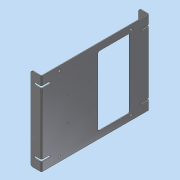
# Autodesk Inventor part: Innengehäuse gebogen
Saved by Autodesk Inventor 2015 SP1 (Build 190203100, 203)
## iProperties
Created: 2015-04-14
Part Number: Innengehäuse gebogen
Material: Stahl AISI 1015
Document SubType Name: Modeling
Designer: ElMatinho
Density: 7.87 g/cm^3
Appearance: Stahl
Author: ElMatinho
Autodesk Inventor part; units mm, degrees
ref_plane "YZ Plane" through (0, 0, 0) normal (1, 0, 0) x (0, 1, 0)
ref_plane "XZ Plane" through (0, 0, 0) normal (0, 1, 0) x (-1, 0, 0)
ref_plane "XY Plane" through (0, 0, 0) normal (0, 0, 1) x (1, 0, 0)
sketch "Skizze1" plane through (0, 0, 0) normal (0, 0, 1) x (1, 0, 0)
  line L0 (-65.8319, 0) -> (313.5681, 0) projected
  line L1 (0, -176.4249) -> (0, 176.4249) projected
  line L2 (13.3681, -123) -> (13.3681, 123)
  line L3 (13.3681, -125.5) -> (259.3681, -125.5) construction
  line L4 (10.8681, 125.5) -> (-11.6319, 125.5)
  line L5 (-11.6319, 125.5) -> (-11.6319, 104.5)
  line L6 (10.8681, -125.5) -> (-11.6319, -125.5)
  line L7 (13.3681, -125.5) -> (35.8681, -125.5) construction
  line L8 (-11.6319, -125.5) -> (-11.6319, -124)
  line L9 (-11.6319, -124) -> (10.8681, -124)
  line L10 (11.8681, -123) -> (11.8681, 123)
  line L11 (10.8681, 124) -> (-10.1319, 124)
  line L12 (-10.1319, 124) -> (-10.1319, 104.5)
  line L13 (-10.1319, 104.5) -> (-11.6319, 104.5)
  arc A0 (13.3681, 123) -> (10.8681, 125.5) centre (10.8681, 123) ccw
  arc A1 (10.8681, -125.5) -> (13.3681, -123) centre (10.8681, -123) ccw
  arc A2 (10.8681, -124) -> (11.8681, -123) centre (10.8681, -123) ccw
  arc A3 (11.8681, 123) -> (10.8681, 124) centre (10.8681, 123) ccw
  point P0 (0, 0)
  point P1 (13.3681, 125.5)
  point P2 (11.8681, -124)
  point P3 (11.8681, 124)
  dimension "d0" = 251
  dimension "d1" = 90
  dimension "d2" = 25
  dimension "d3" = 90
  dimension "d4" = 21
  dimension "d5" = 90
  dimension "d6" = 25
  dimension "d7" = 180
  dimension "d8" = 1.5
  dimension "d9" = 90
  dimension "d10" = 23.5
  dimension "d11" = 90
  dimension "d12" = 248
  dimension "d13" = 90
  dimension "d14" = 22
  dimension "d15" = 90
  dimension "d17" = 1
  constraints: 24 end point, 8 point on circle, 8 point on line, 8 tangent, 6 perpendicular, 4 centre point, 3 parallel, 2 equal length, 2 horizontal, 1 equal radius, 1 vertical
  measures "d0" distance of L3.start point (13.368, 125.5)
  measures "d1" angle of L3 L2
  measures "d2" distance of L4.end point (13.368, 125.5)
  measures "d3" angle of L4 L2
  measures "d4" distance of L4.end L5.end
  measures "d5" angle of L5 L4
  measures "d6" distance of L3.start L6.end
  measures "d7" angle of L6 L7
  measures "d8" distance of L6.end L8.end
  measures "d9" angle of L6 L8
  measures "d10" distance of L8.end point (11.868, -124)
  measures "d11" angle of L8 L9
  measures "d12" distance of point (11.868, -124) point (11.868, 124)
  measures "d13" angle of L10 L9
  measures "d14" distance of L11.end point (11.868, 124)
  measures "d15" angle of L11 L10
  measures "d17" radius of A2
extrude "Extrusion1" add sketch "Skizze1" along normal mid plane 193 contours L10 A3 L11 L1 L4 A0 L2 L0 | L0 L2 A1 L6 L1 L9 A2 L10 | L1 L6 L8 L9 | L11 L12 L13 L5 L4 L1
sketch "Skizze2" plane through (-11.6319, 104.5, 96.5) normal (-1, 0, 0) x (0, 0, 1)
  line L0 (-96.5, -280.2) -> (-96.5, 71.2) projected
  line L1 (-231.6, -104.5) -> (38.6, -104.5) projected
  line L2 (-193, 19.5) -> (-111.5, 19.5)
  line L3 (-111.5, 19.5) -> (-111.5, 0)
  line L4 (-111.5, 0) -> (-193, 0)
  line L5 (-193, 0) -> (-193, 19.5)
  line L6 (-193, -227.5) -> (-193, 18.5) projected
  line L7 (0, 21) -> (-193, 21) projected
  line L8 (0, 19.5) -> (-81.5, 19.5)
  line L9 (-81.5, 19.5) -> (-81.5, 0)
  line L10 (-81.5, 0) -> (0, 0)
  line L11 (0, 0) -> (0, 19.5)
  point P0 (-96.5, -104.5)
  dimension "d20" = 19.5
  dimension "d22" = 1.5
  dimension "d23" = 15
  constraints: 16 end point, 4 symmetric about line, 3 perpendicular, 1 collinear, 1 horizontal
  measures "d20" distance of L4.end L2.start
  measures "d22" distance between parallel lines of L7 L2
  measures "d23" distance between parallel lines of L0 L3
extrude "Extrusion2" cut sketch "Skizze2" against normal blind 2
sketch "Skizze3" plane through (-11.6319, 125.5, 96.5) normal (0, 1, 0) x (1, 0, 0)
  line L0 (-5, 96.5) -> (30, 96.5) projected
  line L1 (11.6319, 231.6) -> (11.6319, -38.6) projected
  line L2 (0, 0) -> (0, 81.5)
  line L3 (0, 81.5) -> (1.5, 81.5)
  line L4 (1.5, 81.5) -> (1.5, 0)
  line L5 (0, 81.5) -> (0, 0) projected
  line L6 (1.5, 0) -> (0, 0)
  line L7 (0, 0) -> (0, 193) projected
  line L8 (22.5, 0) -> (0, 0) projected
  line L9 (0, 193) -> (0, 111.5)
  line L10 (0, 111.5) -> (1.5, 111.5)
  line L11 (1.5, 111.5) -> (1.5, 193)
  line L12 (1.5, 193) -> (0, 193)
  point P0 (11.6319, 96.5)
  dimension "d27" = 1.5
  dimension "d28" = 15
  constraints: 16 end point, 4 symmetric about line, 2 collinear, 2 perpendicular, 1 parallel
  measures "d27" distance of L4.end L2.start
  measures "d28" distance between parallel lines of L0 L3
extrude "Extrusion3" cut sketch "Skizze3" against normal blind 2 contours L7 L12 L11 L10 | L3 L4 L6 L2
fillet "Rundung1" radius 2.5 1 edges at (-11.6319, 125.5, 0)
fillet "Rundung2" radius 1 1 edges at (-10.1319, 124, 0)
hole "Bohrung1" at (-11.6319, 114.5, 0) direction (1, 0, 0) diameter 10 depth 8 tip angle 118
sketch "Skizze4" plane through (13.3681, -123, 96.5) normal (1, 0, 0) x (0, 0, -1)
  line L0 (231.6, 123) -> (-38.6, 123) projected
  line L1 (96.5, -52.7) -> (96.5, 298.7) projected
  line L2 (16, 203.5) -> (177, 203.5)
  line L3 (177, 203.5) -> (177, 128.5)
  line L4 (177, 128.5) -> (16, 128.5)
  line L5 (16, 128.5) -> (16, 203.5)
  line L6 (0, 0) -> (0, 246) projected
  line L7 (193, 0) -> (193, 246) projected
  line L8 (0, 248.5) -> (193, 248.5) projected
  point P0 (96.5, 123)
  dimension "d42" = 16
  dimension "d43" = 75
  dimension "d44" = 16
  dimension "d45" = 45
  constraints: 8 end point, 2 parallel, 1 horizontal, 1 perpendicular
  measures "d42" distance between parallel lines of L6 L5
  measures "d43" distance of L2.end L3.end
  measures "d44" distance between parallel lines of L7 L3
  measures "d45" distance between parallel lines of L8 L2
extrude "Extrusion4" cut sketch "Skizze4" against normal blind 2
hole "Bohrung2" at (13.3681, 83.5, -86.5) direction (-1, 0, 0) diameter 5 depth 8 tip angle 118
pattern_linear "Rechteckige Anordnung1" count 2 spacing 173 along (0, 0, 1) count 2 spacing 167 along (0, -1, 0) of "Bohrung2"
hole "Bohrung3" at (13.3681, -14.5, 29) direction (-1, 0, 0) diameter 2.5 depth 8 tip angle 118
pattern_linear "Rechteckige Anordnung2" count 2 spacing 58 along (0, 0, -1) count 2 spacing 49 along (0, -1, 0) of "Bohrung3"
sketch "Skizze5" plane through (13.3681, -123, 96.5) normal (1, 0, 0) x (0, 0, -1)
  line L0 (96.5, -52.7) -> (96.5, 298.7) projected
  line L1 (231.6, 123) -> (-38.6, 123) projected
  line L2 (20, -2.5) -> (20, 16)
  line L3 (25, -2.5) -> (25, 16)
  arc A0 (25, 16) -> (20, 16) centre (22.5, 16) ccw
  line L4 (0, 0) -> (0, 246) projected
  line L5 (0, -2.5) -> (193, -2.5) projected
  line L6 (20, -2.5) -> (25, -2.5)
  line L7 (173, -2.5) -> (173, 16)
  line L8 (168, -2.5) -> (168, 16)
  arc A1 (173, 16) -> (168, 16) centre (170.5, 16) ccw
  line L9 (173, -2.5) -> (168, -2.5)
  line L10 (20, 248.5) -> (20, 230)
  line L11 (25, 248.5) -> (25, 230)
  arc A2 (20, 230) -> (25, 230) centre (22.5, 230) ccw
  line L12 (20, 248.5) -> (25, 248.5)
  line L13 (173, 248.5) -> (173, 230)
  arc A3 (168, 230) -> (173, 230) centre (170.5, 230) ccw
  line L14 (168, 248.5) -> (168, 230)
  line L15 (173, 248.5) -> (168, 248.5)
  point P0 (96.5, 123)
  point P1 (0, 248.5)
  point P2 (193, 248.5)
  dimension "d78" = 5
  dimension "d79" = 22.5
  dimension "d80" = 18.5
  constraints: 24 end point, 17 symmetric about line, 8 point on circle, 4 centre point, 2 tangent, 2 vertical, 1 collinear, 1 horizontal, 3 other
  measures "d78" diameter of A0
  measures "d79" distance from line of L4 A0.centre
  measures "d80" distance from line of L5 A0.centre
extrude "Extrusion5" cut sketch "Skizze5" against normal blind 5
sketch "Skizze6" plane through (-9.1319, 125.5, -96.5) normal (0, 1, 0) x (1, 0, 0)
  line L0 (9.1319, 38.6) -> (9.1319, -231.6) projected
  line L1 (-7.5, -96.5) -> (27.5, -96.5) projected
  line L2 (7.5, -173) -> (20.5, -173)
  line L3 (21, -177) -> (21, -16) projected
  line L4 (20.5, -173) -> (20.5, -168)
  line L5 (20.5, -168) -> (7.5, -168)
  line L6 (22.5, -193) -> (22.5, -173) projected
  line L7 (17.5, -168) -> (20, -168) projected
  arc A0 (7.5, -168) -> (7.5, -173) centre (7.5, -170.5) ccw
  line L8 (7.5, -20) -> (20.5, -20)
  line L9 (20.5, -20) -> (20.5, -25)
  line L10 (20.5, -25) -> (7.5, -25)
  line L11 (17.5, -25) -> (20, -25)
  arc A1 (7.5, -20) -> (7.5, -25) centre (7.5, -22.5) ccw
  point P0 (9.1319, -96.5)
  dimension "d83" = 5
  dimension "d84" = 2
  dimension "d85" = 15
  constraints: 14 end point, 7 symmetric about line, 4 point on circle, 3 perpendicular, 2 centre point, 2 tangent, 1 collinear, 1 other
  measures "d83" distance of L2.end L4.end
  measures "d84" distance between parallel lines of L6 L4
  measures "d85" distance from line of L6 A0.centre
extrude "Extrusion6" cut sketch "Skizze6" against normal through all
fillet "Rundung3" radius 5 4 edges at (12.6181, 5.5, 80.5) (12.6181, 80.5, 80.5) (12.6181, 80.5, -80.5) (12.6181, 5.5, -80.5)
fillet "Rundung4" radius 5 4 edges at (-10.1319, 124.6456, -96.5) (-11.6319, -124.75, -96.5) (-11.6319, -124.75, 96.5) (-10.1319, 124.6456, 96.5)
